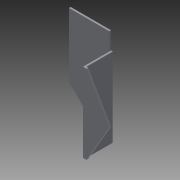
# Autodesk Inventor part: batt-logic support
Saved by Autodesk Inventor 2015 (Build 190159000, 159)
## iProperties
Created: 2015-05-04
Part Number: batt-logic support
Material: Ogólny
Document SubType Name: Modeling
Designer: Kuba
Density: 1 g/cm^3
Appearance: Domyślna
Author: Kuba
Autodesk Inventor part; units mm, degrees
ref_plane "YZ Plane" through (0, 0, 0) normal (1, 0, 0) x (0, 1, 0)
ref_plane "XZ Plane" through (0, 0, 0) normal (0, 1, 0) x (-1, 0, 0)
ref_plane "XY Plane" through (0, 0, 0) normal (0, 0, 1) x (1, 0, 0)
sketch "Szkic1" plane through (0, 0, 0) normal (0, 1, 0) x (-1, 0, 0)
  line L0 (5.9808, -45) -> (10, -45)
  line L1 (10, -45) -> (10, 45)
  line L2 (10, 45) -> (5.9808, 45)
  line L3 (-20, 0) -> (5.9808, -45)
  line L4 (-20, 0) -> (32.0016, 0) construction
  line L5 (-20, 0) -> (5.9808, 45)
  point P0 (0, 0)
  point P1 (-8.1854, 20.4635)
  dimension "d1" = 90
  dimension "d10" = 60
  dimension "d12" = 30
  constraints: 12 end point, 2 horizontal, 1 parallel, 1 perpendicular, 1 point on line, 1 symmetric about line
  measures "d1" distance of L1.end L0.end
  measures "d10" angle of L3 L4
  measures "d12" distance from line of L1 L3.start
extrude "Wyciągnięcie proste1" add sketch "Szkic1" along normal blind 2
sketch "Szkic2" plane through (0, 2, 0) normal (0, 1, 0) x (1, 0, 0)
  line L0 (-10, -45) -> (-8, -45)
  line L1 (-8, -45) -> (-8, 45)
  line L2 (-8, 45) -> (-10, 45)
  line L3 (-10, 45) -> (-10, -45)
  point P0 (0, 0)
  dimension "d4" = 2
  dimension "d13" = 90
  constraints: 8 end point, 2 parallel, 1 horizontal, 1 perpendicular
  measures "d4" distance of L2.end L1.end
  measures "d13" distance of L2.end L0.start
extrude "Wyciągnięcie proste2" add sketch "Szkic2" along normal blind 30
sketch "Szkic3" plane through (-10, 0, -45) normal (-1, 0, 0) x (0, 0, 1)
  line L0 (0, 0) -> (90, 0) projected
  line L1 (90, 0) -> (90, 32) projected
  line L2 (0, 32) -> (90, 32) projected
  line L3 (0, 0) -> (0, 32) projected
  line L4 (90, 0) -> (90, 32) projected
  line L5 (0, 32) -> (90, 32)
  line L6 (90, 32) -> (90, 30)
  line L7 (90, 30) -> (0, 30)
  line L8 (0, 30) -> (0, 32)
  point P0 (45, 0)
  dimension "d7" = 2
  constraints: 8 end point, 2 parallel, 1 horizontal, 1 perpendicular, 1 point on line
  measures "d7" distance of L5.end L6.end
extrude "Wyciągnięcie proste3" add sketch "Szkic3" along normal blind 46 contours L3 L2 L1 L7
sketch "Szkic5" plane through (-10, 0, 45) normal (0, 0, 1) x (1, 0, 0)
  line L0 (0, 0) -> (4.0192, 0) projected
  line L1 (4.0192, 0) -> (4.0192, 2) projected
  line L2 (2, 2) -> (4.0192, 2) projected
  line L3 (2, 2) -> (2, 32) projected
  line L4 (2, 32) -> (-46, 32) projected
  line L5 (-46, 30) -> (-46, 32) projected
  line L6 (0, 30) -> (-46, 30) projected
  line L7 (0, 0) -> (0, 30) projected
  line L8 (-46, 30) -> (0, 30)
  line L9 (0, 30) -> (0, 32)
  line L10 (0, 32) -> (-46, 32)
  line L11 (-46, 32) -> (-46, 30)
  point P0 (10, 0)
  constraints: 8 end point, 2 parallel, 1 horizontal, 1 perpendicular, 1 point on line
extrude "Wyciągnięcie proste4" add sketch "Szkic5" along normal blind 20 contours L6 L5 L4 L9
sketch "Szkic6" plane through (0, 32, 0) normal (0, 1, 0) x (1, 0, 0)
  line L0 (-21.5744, -0.5013) -> (-21.5744, 19.9987) projected
  line L1 (-21.5744, 19.9987) -> (-12.5744, 19.9987) projected
  line L2 (-12.5744, 19.9987) -> (-12.5744, -0.5013) projected
  line L3 (-12.5744, -0.5013) -> (-21.5744, -0.5013) projected
  line L4 (-54, -12.1531) -> (-54, 8.3469) projected
  line L5 (-54, 8.3469) -> (-45, 8.3469) projected
  line L6 (-45, 8.3469) -> (-45, -12.1531) projected
  line L7 (-45, -12.1531) -> (-54, -12.1531) projected
  line L8 (-34.4, 63.5) -> (-34.4, 54.5) projected
  line L9 (-34.4, 54.5) -> (-54.9, 54.5) projected
  line L10 (-54.9, 54.5) -> (-54.9, 63.5) projected
  line L11 (-54.9, 63.5) -> (-34.4, 63.5) projected
  line L12 (-11.9, 63.5) -> (-11.9, 54.5) projected
  line L13 (-11.9, 54.5) -> (-32.4, 54.5) projected
  line L14 (-32.4, 54.5) -> (-32.4, 63.5) projected
  line L15 (-32.4, 63.5) -> (-11.9, 63.5) projected
  line L16 (-34.4, 53.5) -> (-34.4, 44.5) projected
  line L17 (-34.4, 44.5) -> (-54.9, 44.5) projected
  line L18 (-54.9, 44.5) -> (-54.9, 53.5) projected
  line L19 (-54.9, 53.5) -> (-34.4, 53.5) projected
  line L20 (-43.9419, -12.1531) -> (-43.9419, 8.3469) projected
  line L21 (-43.9419, 8.3469) -> (-34.9419, 8.3469) projected
  line L22 (-34.9419, 8.3469) -> (-34.9419, -12.1531) projected
  line L23 (-34.9419, -12.1531) -> (-43.9419, -12.1531) projected
  line L24 (-54.9, 10.5996) -> (-54.9, 40.5996) projected
  line L25 (-54.9, 40.5996) -> (-45.9, 40.5996) projected
  line L26 (-45.9, 40.5996) -> (-45.9, 10.5996) projected
  line L27 (-45.9, 10.5996) -> (-54.9, 10.5996) projected
  circle A0 centre (-16.5, 38.7) radius 1.75 projected
  circle A1 centre (-52.5, -15.3) radius 1.75 projected
  line L28 (-56, -18.8) -> (-10.9, -18.8) projected
  line L29 (-10.9, -18.8) -> (-10.9, 64) projected
  line L30 (-10.9, 64) -> (-56, 64) projected
  line L31 (-56, 64) -> (-56, -18.8) projected
  line L32 (-13.2419, -57.532) -> (-13.2419, -63.753) projected
  line L33 (-13.2419, -63.753) -> (-24.9753, -63.753) projected
  line L34 (-24.9753, -63.753) -> (-24.9753, -57.532) projected
  line L35 (-24.9753, -57.532) -> (-13.2419, -57.532) projected
  line L36 (-18.0913, -22.7408) -> (-18.0913, -28.7314) projected
  line L37 (-18.0913, -28.7314) -> (-30.8017, -28.7314) projected
  line L38 (-30.8017, -28.7314) -> (-30.8017, -22.7408) projected
  line L39 (-30.8017, -22.7408) -> (-18.0913, -22.7408) projected
  line L40 (-13.25, -32.05) -> (-13.25, -55.05) projected
  line L41 (-13.25, -55.05) -> (-29.75, -55.05) projected
  line L42 (-29.75, -55.05) -> (-29.75, -32.05) projected
  line L43 (-29.75, -32.05) -> (-13.25, -32.05) projected
  circle A2 centre (-29, -58.3) radius 1.75 projected
  circle A3 centre (-14, -27.8) radius 1.75 projected
  line L44 (-11, -21.8) -> (-32, -21.8) projected
  line L45 (-32, -21.8) -> (-32, -65.3) projected
  line L46 (-32, -65.3) -> (-11, -65.3) projected
  line L47 (-11, -65.3) -> (-11, -21.8) projected
  line L48 (-35.1226, -33.0908) -> (-35.1226, -40.682) projected
  line L49 (-35.1226, -40.682) -> (-42.292, -40.682) projected
  line L50 (-42.292, -40.682) -> (-42.292, -33.0908) projected
  line L51 (-42.292, -33.0908) -> (-35.1226, -33.0908) projected
  circle A4 centre (-44.2426, -26.4485) radius 3.1458 projected
  line L52 (-51.2011, -28.5045) -> (-51.2011, -38.626) projected
  line L53 (-51.2011, -38.626) -> (-54.1533, -38.626) projected
  line L54 (-54.1533, -38.626) -> (-54.1533, -28.5045) projected
  line L55 (-54.1533, -28.5045) -> (-51.2011, -28.5045) projected
  circle A5 centre (-44.8428, -60.4259) radius 3.3835 projected
  line L56 (-52.6772, -52.7541) -> (-52.6772, -44.1613) projected
  line L57 (-52.6772, -44.1613) -> (-38.391, -44.1613) projected
  line L58 (-38.391, -44.1613) -> (-38.391, -52.7541) projected
  line L59 (-38.391, -52.7541) -> (-52.6772, -52.7541) projected
  circle A6 centre (-53, -58.3) radius 1.5 projected
  circle A7 centre (-38, -28.3) radius 1.5 projected
  line L60 (-35, -21.8) -> (-56, -21.8) projected
  line L61 (-56, -21.8) -> (-56, -65.3) projected
  line L62 (-56, -65.3) -> (-35, -65.3) projected
  line L63 (-35, -65.3) -> (-35, -21.8) projected
  point P0 (0, 0)
hole "Otwór1" at (-53, 32, 58.3) at (-38, 32, 28.3) at (-14, 32, 27.8) at (-29, 32, 58.3) at (-52.5, 32, 15.3) at (-16.5, 32, -38.7) direction (0, -1, 0) diameter 3.5 end through all
